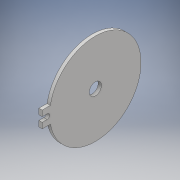
# Autodesk Inventor part: toppart
Saved by Autodesk Inventor 2018 (Build 220112000, 112)
## iProperties
Created: 2019-10-09
Part Number: toppart
Material: 一般
Document SubType Name: Modeling
Designer: Eiji Nishizawa
Density: 1 g/cm^3
Appearance: 既定
Mass: 4.91751 g
Surface Area: 53.5524 cm^2
Volume: 4.91751 cm^3
Author: Eiji Nishizawa
Autodesk Inventor part; units mm, degrees
ref_plane "YZ Plane" through (0, 0, 0) normal (1, 0, 0) x (0, 1, 0)
ref_plane "XZ Plane" through (0, 0, 0) normal (0, 1, 0) x (-1, 0, 0)
ref_plane "XY Plane" through (0, 0, 0) normal (0, 0, 1) x (1, 0, 0)
sketch "スケッチ1" plane through (0, 0, 0) normal (1, 0, 0) x (0, 1, 0)
  circle A0 centre (0, 0) radius 28
  circle A1 centre (0, 0) radius 3.75
  line L0 (-32.55, 5) -> (-27.55, 5)
  line L1 (-27.55, 5) -> (-27.55, -5)
  line L2 (-27.55, -5) -> (-32.55, -5)
  line L3 (-32.55, -5) -> (-32.55, 5)
  line L4 (-32.55, 5) -> (-27.55, -5) construction
  line L5 (-27.55, 5) -> (-32.55, -5) construction
  circle A2 centre (-29.5, 0) radius 1.5
  line L6 (-29.5, 1.5) -> (-32.55, 1.5)
  line L7 (-32.55, 1.5) -> (-32.55, -1.5)
  line L8 (-32.55, -1.5) -> (-29.5, -1.5)
  line L9 (-29.5, -1.5) -> (-29.5, 1.5)
  dimension "d1" = 56
  dimension "d10" = 3
  dimension "d12" = 0
  dimension "d0" = 7.5
  dimension "d2" = 10
  dimension "d3" = 5
  dimension "d11" = 0
  constraints: 20 end point, 4 parallel, 2 coincident, 2 horizontal, 2 perpendicular, 1 centre point, 1 vertical alignment, 5 other
  measures "d0" diameter of A1
  measures "d2" distance of L2.end L0.start
  measures "d3" distance of L1.end L2.end
  measures "d11" distance between parallel lines of L3 L7
extrude "押し出し2" add sketch "スケッチ1" along normal blind 2 contours A0 L1 | L1 A0 | A0 A2 L6 L3 L0 | L2 L3 L8 A2 A0
